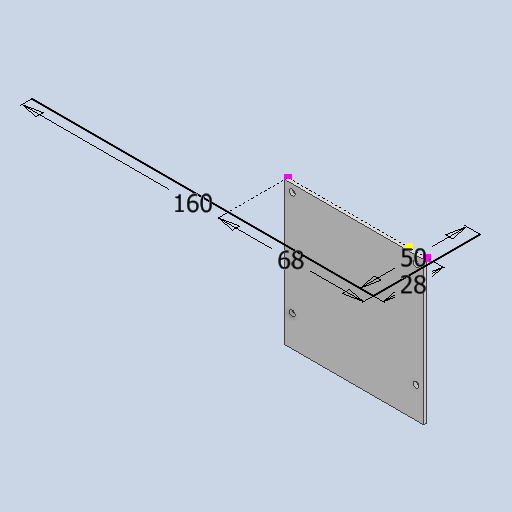
# Autodesk Inventor part: board_rpi
Saved by Autodesk Inventor 2025 (Build 290162000, 162)
## iProperties
Created: 2026-07-21
Part Number: board_rpi
Material: Типовые
Document SubType Name: Modeling
Designer: garin
Density: 1 g/cm^3
Appearance: По умолчанию
Author: garin
Autodesk Inventor part; units mm, degrees
ref_plane "YZ Plane" through (0, 0, 0) normal (1, 0, 0) x (0, 1, 0)
ref_plane "XZ Plane" through (0, 0, 0) normal (0, 1, 0) x (-1, 0, 0)
ref_plane "XY Plane" through (0, 0, 0) normal (0, 0, 1) x (1, 0, 0)
sketch "Эскиз1" plane through (0, 0, 0) normal (0, 0, 1) x (1, 0, 0)
  line L0 (-73.63, -2.23) -> (5.37, -2.23) projected
  arc A0 (5.37, -2.23) -> (8.37, 0.77) centre (5.37, 0.77) ccw projected
  line L1 (8.37, 0.77) -> (8.37, 50.77) projected
  arc A1 (8.37, 50.77) -> (5.37, 53.77) centre (5.37, 50.77) ccw projected
  line L2 (5.37, 53.77) -> (-73.63, 53.77) projected
  arc A2 (-73.63, 53.77) -> (-76.63, 50.77) centre (-73.63, 50.77) ccw projected
  line L3 (-76.63, 50.77) -> (-76.63, 0.77) projected
  arc A3 (-76.63, 0.77) -> (-73.63, -2.23) centre (-73.63, 0.77) ccw projected
  circle A4 centre (4.87, 50.27) radius 1.35 projected
  circle A5 centre (-53.13, 50.27) radius 1.35 projected
  circle A6 centre (0.07, 48.67) radius 0.325 projected
  circle A7 centre (-5.73, 48.67) radius 0.325 projected
  circle A8 centre (-68.88, 49.235) radius 1.65 projected
  circle A9 centre (4.87, 44.27) radius 1.55 projected
  circle A10 centre (-68.88, 37.805) radius 1.65 projected
  circle A11 centre (-53.13, 7.27) radius 1.55 projected
  circle A12 centre (4.87, 1.27) radius 1.35 projected
  circle A13 centre (-53.13, 1.27) radius 1.35 projected
  line L4 (5.37, -2.23) -> (8.37, -2.23) construction
  line L5 (8.37, -2.23) -> (8.37, 0.77) construction
  line L6 (8.37, 0.77) -> (5.37, 0.77) construction
  line L7 (5.37, 0.77) -> (5.37, -2.23) construction
  line L8 (8.37, -2.23) -> (-56.63, -2.23)
  line L9 (-56.63, -2.23) -> (-56.63, 53.77)
  line L10 (-56.63, 53.77) -> (8.37, 53.77)
  line L11 (8.37, 53.77) -> (8.37, -2.23)
  line L12 (8.37, -2.23) -> (-56.63, -2.23)
  line L13 (-56.63, -2.23) -> (-56.63, -13.23)
  line L14 (-56.63, -13.23) -> (8.37, -13.23)
  line L15 (8.37, -13.23) -> (8.37, -2.23)
  line L16 (-56.63, 53.77) -> (8.37, 53.77)
  line L17 (8.37, 53.77) -> (8.37, 61.77)
  line L18 (8.37, 61.77) -> (-56.63, 61.77)
  line L19 (-56.63, 61.77) -> (-56.63, 53.77)
  point P0 (0, 0)
  point P1 (8.37, 0.77)
  point P2 (8.37, 53.77)
  dimension "d0" = 65
  dimension "d1" = 56
  dimension "d8" = 65
  dimension "d9" = 11
  dimension "d10" = 8
  constraints: 32 end point, 8 parallel, 4 horizontal, 4 perpendicular
  measures "d0" distance of L9.end L10.end
  measures "d1" distance of L8.end L9.end
  measures "d8" distance of L14.end L13.end
  measures "d9" distance of L13.end L12.end
  measures "d10" distance of L17.end L16.end
extrude "Выдавливание1" add sketch "Эскиз1" along normal blind 1.5 contours L9 L2 A1 L1 A0 L0 | L0 L8 L15 L14 L13 | A0 L11 L8 | L10 L11 A1 | A6 | A7 | A9 | A11
sketch "Эскиз2" plane through (-56.63, 53.77, 0) normal (0, 1, 0) x (1, 0, 0)
  line L0 (0, 0) -> (65, 0) construction
  line L1 (0, 0) -> (68, 0) construction
  line L2 (68, 0) -> (68, -28) construction
  line L3 (68, -28) -> (0, -28) construction
  line L4 (0, -28) -> (0, 0) construction
  line L5 (68, -28) -> (-92, -28)
  line L6 (68, -28) -> (68, 22)
  point P0 (56.63, 0)
  dimension "d4" = 68
  dimension "d5" = 28
  dimension "d6" = 160
  dimension "d7" = 50
  constraints: 12 end point, 2 horizontal, 2 parallel, 1 perpendicular, 1 vertical
  measures "d4" distance of L2.end L3.end
  measures "d5" distance of L1.end L2.end
  measures "d6" distance of L2.end L5.end
  measures "d7" distance of L2.end L6.end
